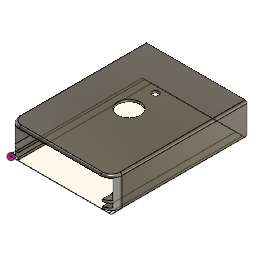
Raspi Shield (Autodesk Fusion 360 design; units mm, degrees)
Autodesk Fusion 360 part; units mm, degrees
sketch "Sketch1" plane through (0, 0, 0) normal (0, 0, 1) x (1, 0, 0)
  line L0 (0, 0) -> (73.6, 0)
  line L1 (73.6, 0) -> (73.6, 100.6)
  line L2 (73.6, 100.6) -> (0, 100.6)
  line L3 (0, 100.6) -> (0, 0)
  line L4 (5.1, 0) -> (68.5, 0)
  line L5 (68.5, 0) -> (68.5, 100.6)
  line L6 (68.5, 100.6) -> (5.1, 100.6)
  line L7 (5.1, 100.6) -> (5.1, 0)
  line L8 (-1.8, 0) -> (75.4, 0)
  line L9 (75.4, 0) -> (75.4, 100.6)
  line L10 (75.4, 100.6) -> (-1.8, 100.6)
  line L11 (-1.8, 100.6) -> (-1.8, 0)
  dimension "d1" = 73.6
  dimension "d2" = 100.6
  dimension "d3" = 63.4
  dimension "d4" = 5.1
  dimension "d6" = 1.8
  dimension "d7" = 1.8
  constraint horizontal L0
  constraint vertical L1
  constraint horizontal L2
  constraint vertical L3
  constraint coincident L0.start L3.end
  constraint horizontal L4
  constraint vertical L5
  constraint horizontal L6
  constraint vertical L7
  constraint collinear L2 L6
  constraint collinear L0 L4
  constraint horizontal L8
  constraint vertical L9
  constraint horizontal L10
  constraint vertical L11
  constraint collinear L6 L10
  constraint collinear L4 L8
  measures "d1" distance of L0.start L0.end
  measures "d2" distance of L0.start L2.end
  measures "d3" distance of L4.start L4.end
  measures "d4" distance of L3 L7
  measures "d6" distance of L3 L11 L0.start
  measures "d7" distance of L1 L9
extrude "Extrude1" add sketch "Sketch1" along normal blind 1.8 contours L0 L2 L3 L7 L8 L10 | L3 L8 L10 L11 | L0 L1 L2 L5 L8 L10 | L1 L8 L9 L10 makes body 1 at (70.8, 33.5333, 0) makes body 2 at (0.5, 67.0667, 0)
extrude "Extrude2" add sketch "Sketch1" along normal blind 4.8 separate body contours L3 L8 L10 L11 | L1 L8 L9 L10 makes body 3 at (-1.8, 67.0667, 1.6) makes body 4 at (75.4, 33.5333, 1.6)
extrude "Extrude3" add sketch "Sketch1" along normal blind 1.8 from surface at 4.8 separate body contours L0 L2 L3 L7 L8 L10 | L3 L8 L10 L11 | L0 L1 L2 L5 L8 L10 | L1 L8 L9 L10 makes body 5 at (70.8, 33.5333, 4.8) makes body 6 at (0.5, 67.0667, 4.8)
extrude "Extrude4" add sketch "Sketch1" along normal blind 16 from surface at 5 separate body contours L3 L8 L10 L11 | L1 L8 L9 L10 makes body 7 at (75.4, 33.5333, 10.3333) makes body 8 at (-1.8, 67.0667, 10.3333)
extrude "Extrude5" add sketch "Sketch1" along normal blind 1.8 from surface at 21 separate body makes body 9
sketch "Sketch2" plane through (0, 100.6, 0) normal (0, 1, 0) x (-1, 0, 0)
  line L0 (-75.4, 21) -> (1.8, 21)
  line L1 (1.8, 21) -> (1.8, 22.8)
  line L2 (1.8, 22.8) -> (-75.4, 22.8)
  line L3 (-75.4, 22.8) -> (-75.4, 21)
  line L4 (-75.4, 0) -> (1.8, 0)
  line L5 (1.8, 0) -> (1.8, 22.8)
  line L6 (1.8, 22.8) -> (-75.4, 22.8)
  line L7 (-75.4, 22.8) -> (-75.4, 0)
  line L8 (1.8, 5) -> (1.8, 21)
  line L9 (-75.4, 5) -> (-75.4, 21)
  line L10 (-75.4, 0) -> (1.8, 0)
  constraint horizontal L4
  constraint vertical L5
  constraint horizontal L6
  constraint vertical L7
  constraint collinear L2 L6
  constraint collinear L5 L8
  constraint collinear L7 L9
  constraint collinear L4 L10
extrude "Extrude6" add sketch "Sketch2" along normal blind 1.8 bodies 1 2 3 4 5 6 7 8 9
fillet "Fillet1" radius 8 2 edges at (-1.8, 0, 11.4) (75.4, 0, 11.4) on bodies 1
fillet "Fillet2" radius 1.5 5 edges at (-1.8, 55.2, 22.8) (0.5431, 2.3431, 22.8) (36.8, 0, 22.8) (73.0569, 2.3431, 22.8) (75.4, 55.2, 22.8) on bodies 1
sketch "Sketch3" plane through (0, 0, 22.8) normal (0, 0, 1) x (-1, 0, 0)
  line L0 (0.3, -102.4) -> (0.3, -8)
  arc A0 (0.3, -8) -> (-6.2, -1.5) centre (-6.2, -8) ccw
  line L1 (-6.2, -1.5) -> (-67.4, -1.5)
  arc A1 (-67.4, -1.5) -> (-73.9, -8) centre (-67.4, -8) ccw
  line L2 (-73.9, -8) -> (-73.9, -102.4)
  line L3 (-73.9, -102.4) -> (0.3, -102.4)
  line L4 (0.3, -102.4) -> (-71.9962, -3.4038) construction
  circle A2 centre (-35.8481, -52.9019) radius 8.5
  line L5 (-35.8481, -72.9019) -> (-35.8481, -52.9019)
  circle A3 centre (-35.8481, -72.9019) radius 2.5
  dimension "d26" = 17
  dimension "d27" = 20
  dimension "d28" = 5
  constraint coincident L0.start L3.end
  constraint midpoint A1 L4.end
  constraint midpoint L4 A2.centre
  constraint coincident A2.centre L5.end
  constraint perpendicular L3 L5
  constraint coincident L5.start A3.centre
  measures "d26" diameter of A2
  measures "d27" distance of L5.start A2.centre
  measures "d28" diameter of A3
extrude "Extrude7" cut sketch "Sketch3" against normal blind 1.8 contours A2 | A3 bodies 1
equation "d4 = ( 10.2 / 2 ) * 1 mm"
equation "t = 1.8 mm" comment "thickness"
equation "d6 = t"
equation "d7 = t"
equation "d8 = t"
equation "d10 = t + 3 mm"
equation "d12 = t + 3 mm"
equation "d13 = t"
equation "ra = 8 mm" comment "radius"
equation "d16 = 2 mm + 3 mm"
equation "d19 = 19 mm + 2 mm"
equation "d20 = t"
equation "d22 = t"
equation "d24 = ra"
equation "d29 = -t"
